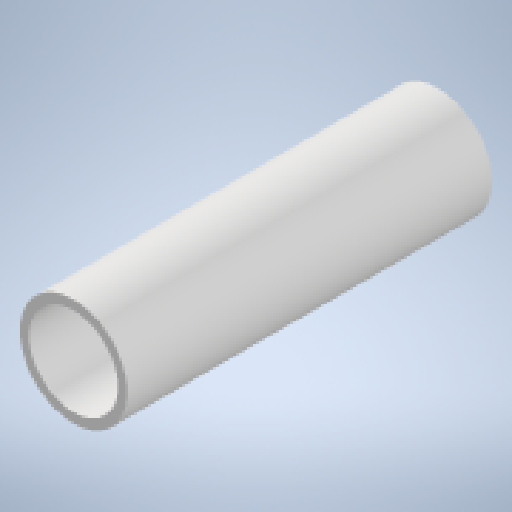
# Autodesk Inventor part: TuboL
Saved by Autodesk Inventor 2023.1 (Build 271208000, 208)
## iProperties
Created: 2022-08-28
Part Number: TuboL
Material: Generic
Document SubType Name: Modeling
Designer: Daniel Peña
Density: 1 g/cm^3
Appearance: Default
Author: Daniel Peña
Autodesk Inventor part; units mm, degrees
ref_plane "YZ Plane" through (0, 0, 0) normal (1, 0, 0) x (0, 1, 0)
ref_plane "XZ Plane" through (0, 0, 0) normal (0, 1, 0) x (-1, 0, 0)
ref_plane "XY Plane" through (0, 0, 0) normal (0, 0, 1) x (1, 0, 0)
sketch "Sketch1" plane through (0, 0, 0) normal (0, 1, 0) x (-1, 0, 0)
  line L0 (0, 30.5885) -> (0, -49.4115)
  line L1 (10.75, 26.0594) -> (8.85, 26.0594)
  line L2 (8.85, 26.0594) -> (8.85, -46.9406)
  line L3 (8.85, -46.9406) -> (10.75, -46.9406)
  line L4 (10.75, -46.9406) -> (10.75, 26.0594)
  point P0 (0, 0)
  dimension "d0" = 80
  dimension "d1" = 17.7
  dimension "d2" = 21.5
  dimension "d3" = 73
  constraints: 10 end point, 2 parallel, 1 horizontal, 1 perpendicular, 1 vertical
  measures "d0" distance of L0.start L0.end
  measures "d1" diameter of L2 L0
  measures "d2" diameter of L4 L0
  measures "d3" distance of L3.end L1.start
revolve "Revolution1" add sketch "Sketch1" angle 360 about axis through (0, 0, 30.5885) along (0, 0, -1)
body "Solid1"
